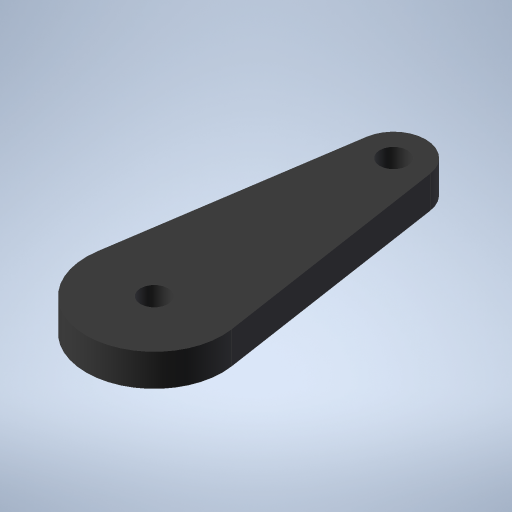
# Autodesk Inventor part: spacing test
Saved by Autodesk Inventor 2024 (Build 280153000, 153)
## iProperties
Created: 2024-04-02
Part Number: spacing test
Material: Generic
Document SubType Name: Modeling
Designer: drew
Density: 1 g/cm^3
Appearance: Default
Author: drew
Autodesk Inventor part; units mm, degrees
ref_plane "YZ Plane" through (0, 0, 0) normal (1, 0, 0) x (0, 1, 0)
ref_plane "XZ Plane" through (0, 0, 0) normal (0, 1, 0) x (-1, 0, 0)
ref_plane "XY Plane" through (0, 0, 0) normal (0, 0, 1) x (1, 0, 0)
sketch "Sketch1" plane through (0, 0, 0) normal (0, 1, 0) x (-1, 0, 0)
  arc A0 (12.5566, -1.9034) -> (-12.5566, -1.9034) centre (0, 0) ccw
  circle A1 centre (0, 0) radius 2.6
  arc A2 (-5.9322, -45.6032) -> (5.9322, -45.6032) centre (0, -44.704) ccw
  circle A3 centre (0, -44.704) radius 2.6
  line L0 (12.5566, -1.9034) -> (5.9322, -45.6032)
  line L1 (-12.5566, -1.9034) -> (-5.9322, -45.6032)
  dimension "d0" = 25.4
  dimension "d5" = 5.2
  dimension "d6" = 12
  dimension "d7" = 44.704
  dimension "d8" = 5.2
  constraints: 4 centre point, 4 end point, 4 point on circle, 4 tangent, 3 coincident, 1 vertical alignment
  measures "d0" diameter of A0
  measures "d5" diameter of A1
  measures "d6" diameter of A2
  measures "d7" distance of point (0, 0) A2.centre
  measures "d8" diameter of A3
extrude "Extrusion1" add sketch "Sketch1" along normal blind 6
body "Solid1"
